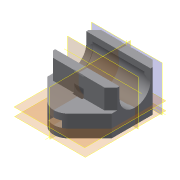
# Autodesk Inventor part: Cycl_soporteRodamientoLinealYV2
Saved by Autodesk Inventor 2015 SP2 (Build 190223200, 223)
## iProperties
Created: 2015-05-07
Material: Genérico
Document SubType Name: Modeling
Designer: E.Beroiz
Density: 1 g/cm^3
Appearance: Valor por defecto
Description: SoporteRodamientoLinealYV2
Author: EDU
Autodesk Inventor part; units mm, degrees
sketch "Boceto1" plane through (0, 0, 0) normal (0, 0, 1) x (1, 0, 0)
  line L0 (-12, 0) -> (12, 0)
  line L1 (15, -3) -> (15, -22.1495)
  line L2 (-15, -22.1495) -> (-15, -3)
  line L3 (12, 0) -> (15, -3)
  line L4 (-12, 0) -> (-15, -3)
  line L5 (-15, -22.1495) -> (-4.9497, -32.1997)
  arc A0 (-4.9497, -32.1997) -> (4.9497, -32.1997) centre (0, -27.25) ccw
  line L6 (4.9497, -32.1997) -> (15, -22.1495)
  point P0 (0, 0)
  point P1 (-15, 0)
  point P2 (15, 0)
  point P3 (0, 0)
  point P4 (0, -34.25)
  point P5 (15, 0)
  point P6 (0, -34.25)
  dimension "d0" = 30
  dimension "d5" = 3
  dimension "d6" = 3
  dimension "d10" = 135
  dimension "d55" = 27.25
  dimension "d59" = 7
  dimension "d60" = 34.25
  constraints: 14 end point, 6 point on line, 3 coincident, 3 point on circle, 2 equal length, 2 perpendicular, 2 tangent, 2 vertical alignment, 1 centre point, 1 horizontal, 1 horizontal alignment, 1 midpoint
  measures "d0" distance of point (-15, 0) point (15, 0)
  measures "d5" distance of L0.end point (15, 0)
  measures "d6" distance of L1.start point (15, 0)
  measures "d10" angle of L2 L5
  measures "d55" distance from line of L0 A0.centre
  measures "d59" radius of A0
  measures "d60" distance from line of point (0, -34.25) L0
extrude "Extrusión1" add sketch "Boceto1" along normal blind 10
sketch "Boceto2" plane through (0, 0, 10) normal (0, 0, 1) x (1, 0, 0)
  line L0 (15, -22.1495) -> (15, -3) projected
  line L1 (15, -3) -> (12, 0) projected
  line L2 (12, 0) -> (-12, 0) projected
  line L3 (-12, 0) -> (-15, -3) projected
  line L4 (-15, -3) -> (-15, -22.1495) projected
  line L5 (-15, -22.1495) -> (-4.9497, -32.1997) projected
  arc A0 (-4.9497, -32.1997) -> (4.9497, -32.1997) centre (0, -27.25) ccw projected
  line L6 (4.9497, -32.1997) -> (15, -22.1495) projected
  line L7 (-15, -19.5) -> (-12, -22.5)
  line L8 (-12, -22.5) -> (12, -22.5)
  line L9 (12, -22.5) -> (15, -19.5)
  point P0 (0, 0)
  dimension "d13" = 3
  dimension "d14" = 3
  dimension "d15" = 3
  dimension "d16" = 3
  dimension "d17" = 22.5
  constraints: 6 end point, 2 point on line, 1 horizontal
  measures "d13" horizontal distance of L8.end L9.end
  measures "d14" horizontal distance of L7.end L7.start
  measures "d15" horizontal distance of L7.start L7.end
  measures "d16" horizontal distance of L8.end L9.end
  measures "d17" distance between parallel lines of L8 L2
extrude "Extrusión2" add sketch "Boceto2" along normal blind 9.25 contours L9 L8 L7 L4 L3 L2 L1 L0
sketch "Boceto3" plane through (15, -22.1495, 0) normal (1, 0, 0) x (0, 0, -1)
  line L0 (-19.25, 2.6495) -> (-19.25, 19.1495) projected
  line L1 (-19.25, 19.1495) -> (-19.25, 2.6495) projected
  line L2 (-19.25, 3.6495) -> (-14.25, 3.6495)
  arc A0 (-14.25, 3.6495) -> (-14.25, 18.1495) centre (-14.25, 10.8995) ccw
  line L3 (-14.25, 18.1495) -> (-19.25, 18.1495)
  point P0 (0, 22.1495)
  point P1 (-7, 10.8995)
  point P2 (-19.25, 10.8995)
  dimension "d20" = 12.25
  dimension "d21" = 14.5
  constraints: 4 end point, 3 point on circle, 2 point on line, 2 tangent, 1 centre point, 1 horizontal, 1 horizontal alignment, 1 midpoint, 1 parallel
  measures "d20" distance from line of L0 point (-7, 10.899)
  measures "d21" distance between parallel lines of L2 L3
extrude "Extrusión3" cut sketch "Boceto3" against normal through all
hole "Agujero1" at (0, -27.25, 0) direction (0, 0, 1) diameter 3.75 depth 8 tip angle 118
ref_plane "Plano de trabajo1" through (0, 0, 4) normal (0, 0, 1) x (1, 0, 0)
sketch "Boceto4" plane through (0, 0, 4) normal (0, 0, 1) x (1, 0, 0)
  circle A0 centre (0, -27.25) radius 1.875 projected
  line L0 (0, -23.6502) -> (3.1175, -25.4501)
  line L1 (3.1175, -25.4501) -> (3.1175, -29.0499)
  line L2 (-3.1175, -29.0499) -> (-3.1175, -25.4501)
  line L3 (-3.1175, -25.4501) -> (0, -23.6502)
  line L4 (-3.1175, -29.0499) -> (-3.1175, -35.0499)
  line L5 (-3.1175, -35.0499) -> (3.1175, -35.0499)
  line L6 (3.1175, -35.0499) -> (3.1175, -29.0499)
  point P0 (0, 0)
  point P1 (0, -27.25)
  dimension "d36" = 6.235
  dimension "d37" = 6
  constraints: 14 end point, 2 perpendicular, 1 coincident, 1 vertical, 1 vertical alignment, 8 other
  measures "d36" distance between parallel lines of L2 L1
  measures "d37" distance of L5.end L1.end
extrude "Extrusión4" cut sketch "Boceto4" along normal blind 3
sketch "Boceto5" plane through (0, 0, 0) normal (1, 0, 0) x (0, 1, 0)
  arc A0 (-18.5, 14.25) -> (-4, 14.25) centre (-11.25, 14.25) ccw projected
  circle A1 centre (-11.25, 16.25) radius 11.5
  circle A2 centre (-11.25, 16.25) radius 13.5
  point P0 (0, 0)
  dimension "d44" = 27
  dimension "d45" = 23
  dimension "d46" = 2
  constraints: 2 centre point, 2 coincident, 1 vertical alignment
  measures "d44" diameter of A2
  measures "d45" diameter of A1
  measures "d46" distance of A0.centre A1.centre
extrude "Extrusión5" cut sketch "Boceto5" along normal mid plane 4.5
sketch "Boceto6" plane through (0, 0, 0) normal (1, 0, 0) x (0, 1, 0)
  line L0 (-18.5, 19.25) -> (-19.5, 19.25) projected
  arc A0 (-18.5, 14.25) -> (-4, 14.25) centre (-11.25, 14.25) ccw projected
  circle A1 centre (-11.25, 14.25) radius 7.6
  point P0 (0, 0)
  dimension "d49" = 15.2
  constraints: 1 centre point, 1 coincident
  measures "d49" diameter of A1
extrude "Extrusión6" cut sketch "Boceto6" along normal mid plane 24.2
ref_plane "Plano de trabajo2" through (15, -11.25, 14.25) normal (0, -1, 0) x (1, 0, 0)
sketch "Boceto7" plane through (15, -11.25, 14.25) normal (0, -1, 0) x (1, 0, 0)
  line L0 (-10.0503, -14.25) -> (0, -14.25) projected
  line L1 (0, -14.25) -> (0, -4.25) projected
  line L2 (-10.0503, -4.25) -> (0, -4.25) projected
  line L3 (-10.0503, -14.25) -> (-10.0503, -4.25) projected
  line L4 (-2.9, -7.6) -> (-2.9, 2.2798) projected
  line L5 (-2.9, 0) -> (-2.9, 0) projected
  line L6 (0, 0) -> (-2.9, 0) projected
  line L7 (0, 0) -> (0, 0) projected
  line L8 (0, 0) -> (-2.9, 0) projected
  line L9 (-2.9, -7.3639) -> (-1.67, -7.2479)
  line L10 (-1.67, -7.2479) -> (-2.9, -7.2479)
  line L11 (-2.9, -7.3639) -> (-2.9, -7.2479)
  point P0 (-15, -14.25)
  dimension "d52" = 0.116
  dimension "d53" = 1.23
  constraints: 6 end point, 2 point on line, 1 collinear, 1 perpendicular
  measures "d52" distance of L9.start L10.end
  measures "d53" distance of L9.end L10.end
revolve "Revolución1" cut sketch "Boceto7" angle 360 about axis through (15, -11.25, 14.25) along (-1, 0, 0) contours L10 L9 L4
mirror "Simetría1" about plane through (0, 0, 0) normal (1, 0, 0) of "Revolución1"
equation "\"d6\" = d5"
